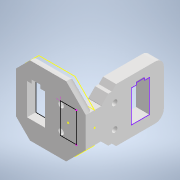
# Autodesk Inventor part: Servo Holder Module
Saved by Autodesk Inventor 2020 (Build 240168000, 168)
## iProperties
Created: 2020-03-03
Part Number: Servo Holder Module
Material: Generic
Document SubType Name: Modeling
Designer: Varun Kumar
Density: 1 g/cm^3
Appearance: Default
Author: Varun Kumar
Autodesk Inventor part; units mm, degrees
ref_plane "YZ Plane" through (0, 0, 0) normal (1, 0, 0) x (0, 1, 0)
ref_plane "XZ Plane" through (0, 0, 0) normal (0, 1, 0) x (-1, 0, 0)
ref_plane "XY Plane" through (0, 0, 0) normal (0, 0, 1) x (1, 0, 0)
sketch "Sketch1" plane through (0, 0, 0) normal (0, 0, 1) x (1, 0, 0)
  line L0 (-38.1, -25.4) -> (38.1, -25.4)
  line L1 (38.1, -25.4) -> (38.1, 25.4)
  line L2 (38.1, 25.4) -> (-38.1, 25.4)
  line L3 (-38.1, 25.4) -> (-38.1, -25.4)
  line L4 (-38.1, -25.4) -> (38.1, 25.4) construction
  line L5 (38.1, -25.4) -> (-38.1, 25.4) construction
  point P0 (0, 0)
  dimension "d0" = 76.2
  dimension "d1" = 50.8
  constraints: 12 end point, 2 midpoint, 2 parallel, 1 horizontal, 1 perpendicular
  measures "d0" distance of L2.end L1.end
  measures "d1" distance of L1.end L0.end
extrude "Extrusion1" add sketch "Sketch1" along normal blind 6.35
sketch "Sketch3" plane through (38.1, -25.4, 0) normal (1, 0, 0) x (0, 0, -1)
  line L0 (0, 0) -> (0, 50.8) projected
  line L1 (0, 50.8) -> (-6.35, 50.8) projected
  line L2 (-6.35, 0) -> (-6.35, 50.8) projected
  line L3 (0, 0) -> (-6.35, 0) projected
  point P0 (0, 25.4)
extrude "Extrusion3" cut sketch "Sketch3" against normal blind 25.4
sketch "Sketch4" plane through (-38.1, -25.4, 0) normal (-1, 0, 0) x (0, 0, 1)
  line L0 (4.925, 17.15) -> (1.425, 17.15)
  line L1 (1.425, 17.15) -> (1.425, 33.65)
  line L2 (1.425, 33.65) -> (4.925, 33.65)
  line L3 (4.925, 33.65) -> (4.925, 17.15)
  line L4 (4.925, 17.15) -> (1.425, 33.65) construction
  line L5 (1.425, 17.15) -> (4.925, 33.65) construction
  point P0 (0, 25.4)
  point P1 (3.175, 25.4)
  dimension "d9" = 3.5
  dimension "d10" = 16.5
  constraints: 12 end point, 2 midpoint, 2 parallel, 1 horizontal, 1 perpendicular
  measures "d9" distance of L1.end L2.end
  measures "d10" distance of L0.end L1.end
extrude "Extrusion4" add sketch "Sketch4" along normal blind 3.302
sketch "Sketch5" plane through (-38.1, -8.25, 4.925) normal (0, 0, 1) x (1, 0, 0)
  line L0 (-3.302, 0) -> (-3.302, 16.5) projected
  line L1 (0, 16.5) -> (0, 0) projected
  line L2 (0, 16.5) -> (-3.302, 16.5) projected
  line L3 (-3.302, 0) -> (-3.302, 16.5) projected
  line L4 (0, 0) -> (-3.302, 0) projected
  line L5 (-3.302, 16.5) -> (-3.175, 16.5)
  line L6 (0, 16.5) -> (-3.302, 16.5) projected
  line L7 (-3.175, 16.5) -> (-3.175, 16.5685)
  line L8 (-3.302, 16.5) -> (-3.302, 0) projected
  line L9 (-3.175, 16.5685) -> (-3.302, 16.5)
  point P0 (38.1, 8.25)
  point P1 (-3.175, 16.5)
  dimension "d13" = 0.127
  constraints: 6 end point, 1 perpendicular, 1 point on line
  measures "d13" distance of L2.end L5.end
sketch3d "3D Sketch1"
  line L0 (-41.402, 8.25, 4.925) -> (-41.402, 8.25, 1.425)
  line L1 (-41.402, 8.25, 1.425) -> (-41.402, -8.25, 1.425)
  line L2 (-41.402, -8.25, 1.425) -> (-41.402, -8.25, 4.925)
  line L3 (-41.402, -8.25, 4.925) -> (-41.402, 8.25, 4.925)
sweep "Sweep1" add profiles "Sketch5" path "3D Sketch1" contours L9 L7 L2
chamfer "Chamfer1" distance 14.2875 angle 45 4 edges at (-38.1, -25.4, 3.175) (-38.1, 25.4, 3.175) (12.7, -25.4, 3.175) (12.7, 25.4, 3.175)
sketch "Sketch6" plane through (-41.402, -25.4, 0) normal (-1, 0, 0) x (0, 0, 1)
  line L0 (-26.5368, -66.9991) -> (26.5368, -66.9991)
  line L1 (26.5368, -66.9991) -> (26.5368, 66.9991)
  line L2 (26.5368, 66.9991) -> (-26.5368, 66.9991)
  line L3 (-26.5368, 66.9991) -> (-26.5368, -66.9991)
  line L4 (0, 0) -> (6.35, 0) projected
  line L5 (-26.5368, -66.9991) -> (26.5368, 66.9991) construction
  line L6 (26.5368, -66.9991) -> (-26.5368, 66.9991) construction
  point P0 (0, 25.4)
  constraints: 12 end point, 2 midpoint, 2 parallel, 1 horizontal, 1 perpendicular
extrude "Extrusion5" cut sketch "Sketch6" against normal blind 28.575
sketch "Sketch7" plane through (0, 0, 0) normal (0, 0, -1) x (-1, 0, 0)
  line L0 (-8.025, 3.175) -> (-8.025, -3.175)
  line L1 (-8.025, -3.175) -> (8.025, -3.175)
  line L2 (8.025, -3.175) -> (8.025, 3.175)
  line L3 (8.025, 3.175) -> (-8.025, 3.175)
  line L4 (-8.025, 4.675) -> (8.025, -1.675) construction
  line L5 (-8.025, -1.675) -> (8.025, 4.675) construction
  line L6 (0, 3.175) -> (0, -3.175)
  point P0 (0, 0)
  point P1 (0, 0)
  dimension "d21" = 6.35
  dimension "d22" = 16.05
  constraints: 14 end point, 2 parallel, 1 midpoint, 1 perpendicular
  measures "d21" distance of L2.end L1.end
  measures "d22" distance of L1.end L0.end
extrude "Extrusion6" add sketch "Sketch7" along normal blind 19.2024
sketch "Sketch9" plane through (0, 0, 6.35) normal (0, 0, 1) x (1, 0, 0)
  line L0 (6.0307, -10.9832) -> (5.9693, 11.0167) projected
  line L1 (-6.0307, 10.9832) -> (6.0307, 10.9832)
  line L2 (6.0307, 10.9832) -> (6.0307, -10.9832)
  line L3 (6.0307, -10.9832) -> (-6.0307, -10.9832)
  line L4 (-6.0307, -10.9832) -> (-6.0307, 10.9832)
  point P0 (0, 0)
  constraints: 8 end point, 2 parallel, 1 horizontal, 1 perpendicular
sketch "Sketch10" plane through (-12.827, -25.4, 0) normal (-1, 0, 0) x (0, 0, 1)
  line L0 (0, 0) -> (0, 50.8) projected
  line L1 (6.35, 0) -> (0, 0) projected
  line L2 (6.35, 50.8) -> (6.35, 0) projected
  line L3 (0, 50.8) -> (6.35, 50.8) projected
  point P0 (0, 25.4)
extrude "Extrusion7" add sketch "Sketch10" along normal blind 25.4
chamfer "Chamfer2" distance 10.16 angle 45 1 edges at (-38.227, 25.4, 3.175)
chamfer "Chamfer3" distance 10.16 angle 45 1 edges at (-38.227, -25.4, 3.175)
sketch "Sketch11" plane through (0, 0, 6.35) normal (0, 0, 1) x (1, 0, 0)
  line L0 (-29.728, 10.9832) -> (-17.6666, 10.9832)
  line L1 (-17.6666, -10.9832) -> (-29.728, -10.9832)
  line L2 (-29.728, -10.9832) -> (-29.728, 10.9832)
  line L3 (-17.6666, -10.9832) -> (-17.6666, 10.9832)
  line L4 (-30.998, 12.2532) -> (-16.3966, 12.2532)
  line L5 (-16.3966, 12.2532) -> (-16.3966, -12.2532)
  line L6 (-16.3966, -12.2532) -> (-30.998, -12.2532)
  line L7 (-30.998, -12.2532) -> (-30.998, 12.2532)
  line L8 (-17.6666, 10.9832) -> (-18.9366, 10.9832)
  line L9 (-29.728, 10.9832) -> (-28.458, 10.9832)
  line L10 (-18.9366, 10.9832) -> (-28.458, 10.9832)
  line L11 (-28.458, 10.9832) -> (-28.458, 15.1856)
  line L12 (-28.458, 15.1856) -> (-18.9366, 15.1856)
  line L13 (-18.9366, 15.1856) -> (-18.9366, 10.9832)
  point P0 (0, 0)
  dimension "d54" = 1.27
  dimension "d55" = 1.27
  dimension "d56" = 1.27
  constraints: 28 end point, 4 parallel, 3 perpendicular, 2 horizontal, 2 point on line, 1 coincident, 3 other
  measures "d54" distance between parallel lines of L2 L7
  measures "d55" distance of L0.end L8.end
  measures "d56" distance of L2.end L9.end
extrude "Extrusion8" cut sketch "Sketch11" against normal up to surface (6.35 mm away) contours L0 L3 L1 L2
sketch "Sketch12" plane through (0, 0, 6.35) normal (0, 0, 1) x (1, 0, 0)
  arc A0 (-5.2182, -6.4143) -> (-5.5402, -10.4006) centre (-5.418, -8.4043) ccw projected
  arc A1 (-5.5402, -10.4006) -> (-5.2182, -6.4143) centre (-5.3404, -8.4106) ccw projected
  arc A2 (-5.3792, 10.6071) -> (-5.3792, 6.6078) centre (-5.418, 8.6074) ccw projected
  arc A3 (-5.3792, 6.6078) -> (-5.3792, 10.6071) centre (-5.3404, 8.6074) ccw projected
  line L0 (-14.078, 16.1258) -> (3.242, 16.1258) projected
  line L1 (-14.078, 16.1258) -> (-14.078, -15.929) projected
  line L2 (-14.078, -15.929) -> (3.242, -15.929) projected
  line L3 (3.242, 16.1258) -> (3.242, -15.929) projected
  circle A4 centre (-5.3404, -8.4106) radius 2
  circle A5 centre (-5.3404, 8.6074) radius 2
  point P0 (0, 0)
  point P1 (-5.3792, 6.6078)
  point P2 (-5.2182, -6.4143)
  point P3 (-5.5402, -10.4006)
  dimension "d38" = 4
  dimension "d39" = 4
  constraints: 2 centre point, 2 coincident
  measures "d38" diameter of A4
  measures "d39" diameter of A5
extrude "Extrusion9" cut sketch "Sketch12" against normal up to surface (6.35 mm away) contours A1 A4 | A3 A5
sketch "Sketch13" plane through (-8.025, 3.175, 0) normal (0, 1, 0) x (1, 0, 0)
  line L0 (16.05, 19.2024) -> (0, 19.2024) projected
  circle A0 centre (8.025, 4.3815) radius 2.25
  circle A1 centre (8.025, 13.1445) radius 2.25
  line L1 (16.05, 0) -> (0, 0) projected
  line L2 (16.05, 0) -> (16.05, 19.2024) projected
  line L3 (0, 19.2024) -> (16.05, 19.2024) projected
  line L4 (0, 0) -> (0, 19.2024) projected
  line L5 (8.025, 0) -> (12.4065, 0)
  line L6 (6.4375, 0) -> (20.725, 0) projected
  line L7 (8.025, 0) -> (8.025, 4.3815)
  line L8 (8.025, 0) -> (12.4065, 0) construction
  line L9 (8.025, 0) -> (21.1695, 0)
  line L10 (8.025, 0) -> (8.025, 13.1445)
  line L11 (16.05, 0) -> (0, 0) projected
  line L12 (8.025, 0) -> (21.1695, 0) construction
  dimension "d44" = 4.5
  dimension "d45" = 4.5
  dimension "d48" = 4.3815
  dimension "d49" = 4.3815
  dimension "d50" = 90
  dimension "d51" = 13.1445
  dimension "d52" = 13.1445
  dimension "d53" = 90
  constraints: 12 end point, 3 perpendicular, 2 centre point, 2 coincident, 2 horizontal, 2 point on line
  measures "d44" diameter of A0
  measures "d45" diameter of A1
  measures "d48" distance of L5.start L5.end
  measures "d49" distance of L5.start L7.end
  measures "d50" angle of L8 L7
  measures "d51" distance of L5.start L9.end
  measures "d52" distance of L5.start L10.end
  measures "d53" angle of L12 L10
extrude "Extrusion10" cut sketch "Sketch13" against normal up to surface (6.35 mm away) contours A1 | A0 L10 L7 | L7 L10 A0
sketch "Sketch14" plane through (0, 0, -19.2024) normal (0, 0, -1) x (-1, 0, 0)
  line L0 (8.025, 3.175) -> (8.025, -3.175) projected
  line L1 (-8.025, -3.175) -> (-8.025, 3.175) projected
  line L2 (8.025, 3.175) -> (-8.025, 3.175)
  line L3 (-8.025, 3.175) -> (-8.025, -3.175)
  line L4 (-8.025, -3.175) -> (8.025, -3.175)
  line L5 (8.025, -3.175) -> (8.025, 3.175)
  point P0 (0, 0)
  constraints: 8 end point, 2 parallel, 1 horizontal, 1 perpendicular
sketch "Sketch16" plane through (0, 0, 6.35) normal (0, 0, 1) x (1, 0, 0)
  line L0 (-29.728, -10.9832) -> (-29.728, 10.9832) projected
  line L1 (-17.6666, -10.9832) -> (-29.728, -10.9832) projected
  line L2 (-17.6666, 10.9832) -> (-17.6666, -10.9832) projected
  line L3 (-29.728, 10.9832) -> (-17.6666, 10.9832) projected
  line L4 (-29.982, -11.2372) -> (-29.982, 11.2372)
  line L5 (-29.982, 11.2372) -> (-17.4126, 11.2372)
  line L6 (-17.4126, 11.2372) -> (-17.4126, -11.2372)
  line L7 (-17.4126, -11.2372) -> (-29.982, -11.2372)
  point P0 (0, 0)
  dimension "d62" = 0.254
  constraints: 8 end point, 3 other
  measures "d62" distance between parallel lines of L1 L7
extrude "Extrusion12" cut sketch "Sketch16" against normal up to surface (6.35 mm away)
sketch "Sketch17" plane through (0, 0, 6.35) normal (0, 0, 1) x (1, 0, 0)
  line L0 (-17.4126, 11.2372) -> (-29.982, 11.2372) projected
  line L1 (-29.982, 11.2372) -> (-26.807, 11.2372)
  line L2 (-17.4126, 11.2372) -> (-20.5876, 11.2372)
  line L3 (-26.807, 11.2372) -> (-20.5876, 11.2372)
  line L4 (-20.5876, 11.2372) -> (-20.5876, 12.8247)
  line L5 (-20.5876, 12.8247) -> (-26.807, 12.8247)
  line L6 (-26.807, 12.8247) -> (-26.807, 11.2372)
  point P0 (0, 0)
  dimension "d65" = 3.175
  dimension "d66" = 3.175
  dimension "d67" = 1.5875
  constraints: 12 end point, 2 parallel, 2 point on line, 1 horizontal, 1 perpendicular
  measures "d65" distance of L0.end L1.end
  measures "d66" distance of L0.start L2.end
  measures "d67" distance of L4.end L3.end
extrude "Extrusion13" cut sketch "Sketch17" against normal up to surface (6.35 mm away)
sketch "Sketch18" plane through (0, 0, -19.2024) normal (0, 0, -1) x (-1, 0, 0)
  line L0 (8.025, -3.175) -> (8.025, 3.175) projected
  line L1 (8.025, 3.175) -> (-8.025, 3.175) projected
  line L2 (-8.025, 3.175) -> (-8.025, -3.175) projected
  line L3 (-8.025, -3.175) -> (8.025, -3.175) projected
  line L4 (8.025, -3.175) -> (8.025, 3.175) projected
  line L5 (8.025, 3.175) -> (-8.025, 3.175) projected
  line L6 (-8.025, 3.175) -> (-8.025, -3.175) projected
  line L7 (-8.025, -3.175) -> (8.025, -3.175) projected
  point P0 (0, 0)
extrude "Extrusion14" cut sketch "Sketch18" against normal up to surface (19.2024 mm away)
sketch "Sketch19" plane through (0, 0, 0) normal (0, 0, -1) x (-1, 0, 0)
  line L0 (38.227, -15.24) -> (28.067, -25.4) projected
  line L1 (38.227, 15.24) -> (38.227, -15.24) projected
  line L2 (28.067, 25.4) -> (38.227, 15.24) projected
  line L3 (1.5875, 25.4) -> (28.067, 25.4) projected
  line L4 (-12.7, 11.1125) -> (1.5875, 25.4) projected
  line L5 (-12.7, 11.1125) -> (-12.7, -11.1125) projected
  line L6 (1.5875, -25.4) -> (-12.7, -11.1125) projected
  line L7 (28.067, -25.4) -> (1.5875, -25.4) projected
  circle A0 centre (5.3404, -8.4106) radius 2 projected
  circle A1 centre (5.3404, 8.6074) radius 2 projected
  line L8 (20.5876, 11.2372) -> (20.5876, 12.8247) projected
  line L9 (20.5876, 12.8247) -> (26.807, 12.8247) projected
  line L10 (26.807, 12.8247) -> (26.807, 11.2372) projected
  line L11 (26.807, 11.2372) -> (29.982, 11.2372) projected
  line L12 (29.982, 11.2372) -> (29.982, -11.2372) projected
  line L13 (29.982, -11.2372) -> (17.4126, -11.2372) projected
  line L14 (17.4126, -11.2372) -> (17.4126, 11.2372) projected
  line L15 (17.4126, 11.2372) -> (20.5876, 11.2372) projected
  line L16 (-12.7, -11.1125) -> (-3.175, -11.1125)
  line L17 (-3.175, -11.1125) -> (-3.175, 11.1125)
  line L18 (-3.175, 11.1125) -> (-12.7, 11.1125)
  line L19 (-12.7, 11.1125) -> (-12.7, -11.1125)
  point P0 (0, 0)
  dimension "d72" = 9.525
  constraints: 8 end point, 2 parallel, 1 horizontal, 1 perpendicular
  measures "d72" distance of L18.end L17.end
extrude "Extrusion15" add sketch "Sketch19" along normal blind 12.7 contours L5 L18 L17 L16
sketch "Sketch20" plane through (0, 0, -12.7) normal (0, 0, -1) x (-1, 0, 0)
  line L0 (-12.7, -11.1125) -> (-3.175, -11.1125) projected
  line L1 (-3.175, -11.1125) -> (-3.175, 11.1125) projected
  line L2 (-3.175, 11.1125) -> (-12.7, 11.1125) projected
  line L3 (-12.7, 11.1125) -> (-12.7, -11.1125) projected
  line L4 (-3.175, -19.648) -> (-12.7, -19.648)
  line L5 (-12.7, -19.648) -> (-12.7, 19.648)
  line L6 (-12.7, 19.648) -> (-3.175, 19.648)
  line L7 (-3.175, 19.648) -> (-3.175, -19.648)
  line L8 (-3.175, -19.648) -> (-12.7, 19.648) construction
  line L9 (-12.7, -19.648) -> (-3.175, 19.648) construction
  point P0 (0, 0)
  point P1 (-7.9375, 0)
  constraints: 12 end point, 2 midpoint, 2 parallel, 1 horizontal, 1 perpendicular
extrude "Extrusion16" add sketch "Sketch20" along normal blind 38.1
sketch "Sketch21" plane through (0, 0, 0) normal (0, 0, -1) x (-1, 0, 0)
  line L0 (29.982, -11.2372) -> (17.4126, -11.2372) projected
  line L1 (29.982, -11.2372) -> (17.4126, -11.2372)
  line L2 (17.4126, -11.2372) -> (17.4126, -11.7372)
  line L3 (17.4126, -11.7372) -> (29.982, -11.7372)
  line L4 (29.982, -11.7372) -> (29.982, -11.2372)
  line L5 (29.982, -11.7372) -> (30.232, -11.7372)
  line L6 (30.232, -11.7372) -> (30.232, 11.2372)
  line L7 (30.232, 11.2372) -> (29.982, 11.2372)
  line L8 (29.982, 11.2372) -> (29.982, -11.7372)
  line L9 (17.4126, -11.7372) -> (17.1626, -11.7372)
  line L10 (17.1626, -11.7372) -> (17.1626, 11.2372)
  line L11 (17.1626, 11.2372) -> (17.4126, 11.2372)
  line L12 (17.4126, 11.2372) -> (17.4126, -11.7372)
  point P0 (0, 0)
  dimension "d77" = 0.5
  dimension "d78" = 0.25
  dimension "d79" = 0.25
  constraints: 24 end point, 6 parallel, 3 horizontal, 3 perpendicular, 1 point on line
  measures "d77" distance of L2.end L1.end
  measures "d78" distance of L7.end L6.end
  measures "d79" distance of L10.end L11.end
extrude "Extrusion17" cut sketch "Sketch21" against normal up to surface (6.35 mm away)
chamfer "Chamfer4" distance 3.175 angle 45 2 edges at (7.9375, 19.648, -12.7) (7.9375, -19.648, -12.7)
fillet "Fillet2" radius 6.35 2 edges at (7.9375, -19.648, -50.8) (7.9375, 19.648, -50.8)
sketch "Sketch22" plane through (0, 0, 0) normal (0, 0, -1) x (-1, 0, 0)
  line L0 (-12.7, 11.1125) -> (-3.175, 11.1125) projected
  line L1 (-3.175, 11.1125) -> (-3.175, -11.1125) projected
  line L2 (-3.175, -11.1125) -> (-12.7, -11.1125) projected
  line L3 (1.5875, -25.4) -> (-12.7, -11.1125) projected
  line L4 (28.067, -25.4) -> (1.5875, -25.4) projected
  line L5 (38.227, -15.24) -> (28.067, -25.4) projected
  line L6 (38.227, 15.24) -> (38.227, -15.24) projected
  line L7 (28.067, 25.4) -> (38.227, 15.24) projected
  line L8 (1.5875, 25.4) -> (28.067, 25.4) projected
  line L9 (-12.7, 11.1125) -> (1.5875, 25.4) projected
  circle A0 centre (5.3404, -8.4106) radius 2 projected
  circle A1 centre (5.3404, 8.6074) radius 2 projected
  line L10 (26.807, 11.2372) -> (30.232, 11.2372) projected
  line L11 (30.232, 11.2372) -> (30.232, -11.7372) projected
  line L12 (30.232, -11.7372) -> (17.1626, -11.7372) projected
  line L13 (17.1626, -11.7372) -> (17.1626, 11.2372) projected
  line L14 (17.1626, 11.2372) -> (20.5876, 11.2372) projected
  line L15 (20.5876, 11.2372) -> (20.5876, 12.8247) projected
  line L16 (20.5876, 12.8247) -> (26.807, 12.8247) projected
  line L17 (26.807, 12.8247) -> (26.807, 11.2372) projected
  line L18 (26.807, 11.2372) -> (30.232, 11.2372)
  line L19 (30.232, 11.2372) -> (26.807, 11.2372) projected
  line L20 (30.232, -11.7372) -> (30.232, 11.2372) projected
  line L21 (30.232, 11.2372) -> (30.232, -11.7372)
  line L22 (30.232, -11.7372) -> (17.1626, -11.7372) projected
  line L23 (30.232, -11.7372) -> (17.1626, -11.7372)
  line L24 (17.1626, -11.7372) -> (17.1626, 11.2372)
  line L25 (20.5876, 11.2372) -> (17.1626, 11.2372)
  line L26 (20.5876, 11.2372) -> (20.5876, 12.8247) projected
  line L27 (20.5876, 11.2372) -> (20.5876, 12.8247)
  line L28 (20.5876, 12.8247) -> (26.807, 12.8247)
  line L29 (26.807, 11.2372) -> (26.807, 12.8247) projected
  line L30 (26.807, 11.2372) -> (26.807, 12.8247)
  point P0 (0, 0)
  constraints: 16 end point, 5 perpendicular, 1 collinear, 1 horizontal, 1 vertical
sketch "Sketch23" plane through (12.7, -25.4, 0) normal (1, 0, 0) x (0, 0, -1)
  line L0 (36.6513, 37.1926) -> (40.3263, 37.1926)
  line L1 (40.3263, 37.1926) -> (40.3263, 13.7182)
  line L2 (40.3263, 13.7182) -> (26.7569, 13.7182)
  line L3 (26.7569, 13.7182) -> (26.7569, 37.1926)
  line L4 (30.4319, 37.1926) -> (26.7569, 37.1926)
  line L5 (30.4319, 37.1926) -> (30.4319, 38.7801)
  line L6 (30.4319, 38.7801) -> (36.6513, 38.7801)
  line L7 (36.6513, 37.1926) -> (36.6513, 38.7801)
  point P0 (0, 25.4)
  constraints: 16 end point, 2 perpendicular, 1 horizontal, 1 vertical
sketch "Sketch24" plane through (12.7, -25.4, 0) normal (1, 0, 0) x (0, 0, -1)
  arc A0 (50.8, 38.698) -> (44.45, 45.048) centre (44.45, 38.698) ccw projected
  line L0 (15.875, 45.048) -> (44.45, 45.048) projected
  line L1 (12.7, 41.873) -> (15.875, 45.048) projected
  line L2 (12.7, 41.873) -> (12.7, 36.5125) projected
  line L3 (0, 36.5125) -> (12.7, 36.5125) projected
  line L4 (-6.35, 36.5125) -> (0, 36.5125) projected
  line L5 (-6.35, 14.2875) -> (-6.35, 36.5125) projected
  line L6 (0, 14.2875) -> (-6.35, 14.2875) projected
  line L7 (0, 14.2875) -> (12.7, 14.2875) projected
  line L8 (12.7, 14.2875) -> (12.7, 8.927) projected
  line L9 (15.875, 5.752) -> (12.7, 8.927) projected
  line L10 (15.875, 5.752) -> (44.45, 5.752) projected
  arc A1 (44.45, 5.752) -> (50.8, 12.102) centre (44.45, 12.102) ccw projected
  line L11 (50.8, 38.698) -> (50.8, 12.102) projected
  line L12 (63.6753, 38.7801) -> (57.4559, 38.7801)
  line L13 (57.4559, 38.7801) -> (57.4559, 39.7801)
  line L14 (57.4559, 39.7801) -> (63.6753, 39.7801)
  line L15 (63.6753, 39.7801) -> (63.6753, 38.7801)
  point P0 (0, 25.4)
  dimension "d88" = 1
  constraints: 8 end point, 2 parallel, 1 horizontal, 1 perpendicular
  measures "d88" distance of L12.end L13.end
extrude "Extrusion19" cut sketch "Sketch24" against normal up to surface (9.525 mm away) contours L12 L13 L14 L15
sketch "Sketch25" plane through (0, 0, 0) normal (0, 0, -1) x (-1, 0, 0)
  line L0 (-12.7, 11.1125) -> (-3.175, 11.1125) projected
  line L1 (-3.175, 11.1125) -> (-3.175, -11.1125) projected
  line L2 (-3.175, -11.1125) -> (-12.7, -11.1125) projected
  line L3 (1.5875, -25.4) -> (-12.7, -11.1125) projected
  line L4 (28.067, -25.4) -> (1.5875, -25.4) projected
  line L5 (38.227, -15.24) -> (28.067, -25.4) projected
  line L6 (38.227, 15.24) -> (38.227, -15.24) projected
  line L7 (28.067, 25.4) -> (38.227, 15.24) projected
  line L8 (1.5875, 25.4) -> (28.067, 25.4) projected
  line L9 (-12.7, 11.1125) -> (1.5875, 25.4) projected
  circle A0 centre (5.3404, -8.4106) radius 2 projected
  circle A1 centre (5.3404, 8.6074) radius 2 projected
  line L10 (26.807, 11.2372) -> (30.232, 11.2372) projected
  line L11 (30.232, 11.2372) -> (30.232, -11.7372) projected
  line L12 (30.232, -11.7372) -> (17.1626, -11.7372) projected
  line L13 (17.1626, -11.7372) -> (17.1626, 11.2372) projected
  line L14 (17.1626, 11.2372) -> (20.5876, 11.2372) projected
  line L15 (20.5876, 11.2372) -> (20.5876, 12.8247) projected
  line L16 (20.5876, 12.8247) -> (26.807, 12.8247) projected
  line L17 (26.807, 12.8247) -> (26.807, 11.2372) projected
  line L18 (20.5876, 12.8247) -> (26.807, 12.8247)
  line L19 (26.807, 12.8247) -> (26.807, 13.8247)
  line L20 (26.807, 13.8247) -> (20.5876, 13.8247)
  line L21 (20.5876, 13.8247) -> (20.5876, 12.8247)
  point P0 (0, 0)
  dimension "d91" = 1
  constraints: 8 end point, 2 parallel, 1 horizontal, 1 perpendicular
  measures "d91" distance of L19.end L18.end
extrude "Extrusion20" cut sketch "Sketch25" against normal up to surface (6.35 mm away) contours L16 L21 L20 L19
fillet "Fillet4" radius 4.699 7 edges at (-14.8273, -25.4, 0) (-33.147, -20.32, 0) (-38.227, 0, 0) (-33.147, 20.32, 0) (-14.8272, 25.4, 0) (5.5563, 18.2563, 0) (5.5563, -18.2563, 0)
sketch "Sketch26" plane through (0, 0, 0) normal (0, 0, -1) x (-1, 0, 0)
  line L0 (20.5876, 11.2372) -> (20.5876, 13.8247) projected
  line L1 (20.5876, 13.8247) -> (26.807, 13.8247) projected
  line L2 (26.807, 13.8247) -> (26.807, 11.2372) projected
  line L3 (26.807, 11.2372) -> (30.232, 11.2372) projected
  line L4 (30.232, 11.2372) -> (30.232, -11.7372) projected
  line L5 (30.232, -11.7372) -> (17.1626, -11.7372) projected
  line L6 (17.1626, -11.7372) -> (17.1626, 11.2372) projected
  line L7 (17.1626, 11.2372) -> (20.5876, 11.2372) projected
  circle A0 centre (5.3404, 8.6074) radius 2 projected
  circle A1 centre (5.3404, -8.4106) radius 2 projected
  line L8 (3.5339, -20.701) -> (-6.0546, -11.1125) projected
  line L9 (26.1206, -20.701) -> (3.5339, -20.701) projected
  line L10 (33.528, -13.2936) -> (26.1206, -20.701) projected
  line L11 (33.528, 13.2936) -> (33.528, -13.2936) projected
  line L12 (26.1206, 20.701) -> (33.528, 13.2936) projected
  line L13 (3.5339, 20.701) -> (26.1206, 20.701) projected
  line L14 (-6.0546, 11.1125) -> (3.5339, 20.701) projected
  line L15 (-3.175, 11.1125) -> (-3.175, -11.1125) projected
  line L16 (26.807, 13.8247) -> (20.5876, 13.8247) projected
  line L17 (20.5876, 13.8247) -> (26.807, 13.8247)
  line L18 (26.807, 13.8247) -> (26.807, 11.2372)
  line L19 (26.807, 11.2372) -> (30.232, 11.2372)
  line L20 (30.232, 11.2372) -> (30.232, -11.7372) projected
  line L21 (30.232, 11.2372) -> (30.232, -11.7372)
  line L22 (17.1626, -11.7372) -> (30.232, -11.7372) projected
  line L23 (30.232, -11.7372) -> (17.1626, -11.7372)
  line L24 (17.1626, -11.7372) -> (17.1626, 11.2372)
  line L25 (20.5876, 11.2372) -> (17.1626, 11.2372) projected
  line L26 (17.1626, 11.2372) -> (20.5876, 11.2372)
  line L27 (20.5876, 11.2372) -> (20.5876, 13.8247)
  line L28 (-6.0546, 11.1125) -> (-3.175, 11.1125) projected
  line L29 (-3.175, -11.1125) -> (-6.0546, -11.1125) projected
  point P0 (0, 0)
  constraints: 16 end point, 3 collinear, 3 perpendicular, 2 horizontal
sketch "Sketch27" plane through (12.7, -25.4, 0) normal (1, 0, 0) x (0, 0, -1)
  line L0 (30.232, 39.3866) -> (36.4514, 39.3866)
  line L1 (36.4514, 39.3866) -> (36.4514, 36.7991)
  line L2 (36.4514, 36.7991) -> (39.8764, 36.7991)
  line L3 (39.8764, 36.7991) -> (39.8764, 13.8247)
  line L4 (39.8764, 13.8247) -> (26.807, 13.8247)
  line L5 (26.807, 13.8247) -> (26.807, 36.7991)
  line L6 (26.807, 36.7991) -> (30.232, 36.7991)
  line L7 (30.232, 36.7991) -> (30.232, 39.3866)
  point P0 (0, 25.4)
  constraints: 16 end point, 3 perpendicular, 2 horizontal
extrude "Extrusion21" cut sketch "Sketch27" against normal up to surface (9.525 mm away)
sketch "Sketch29" plane through (12.7, -25.4, 0) normal (1, 0, 0) x (0, 0, -1)
  circle A0 centre (14.7694, 33.7421) radius 2
  circle A1 centre (14.7694, 16.7241) radius 2
  point P0 (0, 25.4)
  constraints: 2 centre point, 4 other
extrude "Extrusion23" cut sketch "Sketch29" against normal up to surface (9.525 mm away)
sketch "Sketch30" plane through (0, 0, -12.7) normal (0, 0, 1) x (1, 0, 0)
  line L0 (3.175, 16.473) -> (12.7, 16.473) projected
  line L1 (3.175, 11.1125) -> (3.175, 16.473) projected
  line L2 (3.175, 11.1125) -> (12.7, 11.1125) projected
  line L3 (12.7, 16.473) -> (12.7, 11.1125) projected
  line L4 (12.7, -16.473) -> (3.175, -16.473) projected
  line L5 (12.7, -11.1125) -> (12.7, -16.473) projected
  line L6 (12.7, -11.1125) -> (3.175, -11.1125) projected
  line L7 (3.175, -16.473) -> (3.175, -11.1125) projected
  point P0 (0, 0)
extrude "Extrusion24" add sketch "Sketch30" along normal blind 7.62
chamfer "Chamfer5" distance 5.0165 angle 45 1 edges at (7.9375, -16.473, -5.08)
chamfer "Chamfer6" distance 5.0165 angle 45 1 edges at (7.9375, 16.473, -5.08)
body "Solid1"
